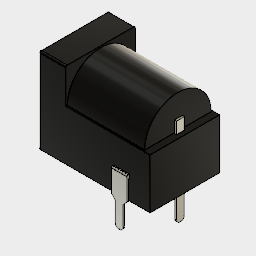
373 Breadboard Friendly 2.1 mm Barrel Jack (Autodesk Fusion 360 design; units mm, degrees)
Autodesk Fusion 360 part; units mm, degrees
sketch "Sketch1" plane through (0, 0, 0) normal (0, 0, 1) x (1, 0, 0)
  line L0 (0, 0) -> (0, 4.5)
  line L1 (0, 4.5) -> (-3.5, 4.5)
  line L2 (-3.5, 4.5) -> (-3.5, -4.5)
  line L3 (-3.5, -4.5) -> (0, -4.5)
  line L4 (0, -4.5) -> (0, 0)
  line L5 (0, 4.5) -> (10.9, 4.5)
  line L6 (10.9, 4.5) -> (10.9, -4.5)
  line L7 (10.9, -4.5) -> (0, -4.5)
  line L8 (0, -4.5) -> (0, 4.5)
  dimension "d1" = 4.5
  dimension "d2" = 3.5
  dimension "d3" = 9
  dimension "d4" = 10.9
  dimension "d5" = 9
  measures "d1" distance of L0.start L0.end
  measures "d2" distance of L0.end L1.end
  measures "d3" distance of L1.end L2.end
  measures "d4" distance of L0.end L5.end
  measures "d5" distance of L0.end L3.end
extrude "Extrude1" add sketch "Sketch1" along normal blind 6.5 contours L0 L4 L5 L6 L7 L8 makes body 1
extrude "Extrude2" add sketch "Sketch1" along normal blind 11 contours L0 L1 L2 L3 L4 L8 bodies 1
sketch "Sketch2" plane through (-3.5, 0, 0) normal (-1, 0, 0) x (0, -1, 0)
  line L0 (-4.5, 0) -> (4.5, 0)
  line L1 (4.5, 0) -> (4.5, 11)
  line L2 (4.5, 11) -> (-4.5, 11)
  line L3 (-4.5, 11) -> (-4.5, 0)
  line L4 (0, 11) -> (0, 0) construction
  line L5 (-4.5, 6.5) -> (4.5, 6.5) construction
  circle A0 centre (0, 6.5) radius 4.3
  circle A1 centre (0, 6.5) radius 3.25
  circle A2 centre (0, 6.472) radius 1
  dimension "d10" = 8.6
  dimension "d11" = 6.5
  dimension "d14" = 2
  measures "d10" diameter of A0
  measures "d11" diameter of A1
  measures "d14" diameter of A2
extrude "Extrude3" add sketch "Sketch2" against normal blind 13.5 contours A0 | A1 | A2 bodies 1
extrude "Extrude4" cut sketch "Sketch2" against normal blind 5 contours A1 bodies 1
sketch "Sketch3" plane through (0, 0, 0) normal (0, 0, 1) x (1, 0, 0)
  line L0 (4.325, -0.5) -> (4.075, -0.5)
  line L1 (4.075, -0.5) -> (4.075, 0.5)
  line L2 (4.075, 0.5) -> (4.325, 0.5)
  line L3 (4.325, 0.5) -> (4.325, -0.5)
  line L4 (4.325, -0.5) -> (4.075, 0.5) construction
  line L5 (4.075, -0.5) -> (4.325, 0.5) construction
  line L6 (3.325, 0.5) -> (3.325, -0.5)
  line L7 (-3.5, 4.5) -> (-3.5, -4.5)
  line L8 (10.325, -0.5) -> (10.075, -0.5)
  line L9 (10.075, -0.5) -> (10.075, 0.5)
  line L10 (10.075, 0.5) -> (10.325, 0.5)
  line L11 (10.325, 0.5) -> (10.325, -0.5)
  line L12 (10.325, -0.5) -> (10.075, 0.5) construction
  line L13 (10.075, -0.5) -> (10.325, 0.5) construction
  point P0 (4.2, 0)
  point P1 (10.2, 0)
  dimension "d17" = 0.25
  dimension "d18" = 1
  dimension "d19" = 1
  dimension "d20" = 7.7
  dimension "d21" = 1
  dimension "d22" = 0.25
  dimension "d23" = 6
  measures "d17" distance of L1.end L2.end
  measures "d18" distance of L0.end L1.end
  measures "d19" distance of L3
  measures "d20" distance of P0 L7
  measures "d21" distance of L8.end L9.end
  measures "d22" distance of L9.end L10.end
  measures "d23" distance of P0 P1
extrude "Extrude11" cut sketch "Sketch3" along normal blind 10 contours L8 L9 L10 L11 bodies 1
extrude "Extrude5" add sketch "Sketch3" along normal blind 8 and the other way blind 3.5 separate body makes body 2 at (4.325, -0.1667, 4.1667) makes body 3 at (10.325, -0.1667, 4.1667)
sketch "Sketch4" plane through (0, -4.5, 0) normal (0, -1, 0) x (1, 0, 0)
  line L0 (-3.5, 0) -> (10.9, 0)
  line L1 (10.9, 0) -> (10.9, 6.5)
  line L2 (10.9, 6.5) -> (0, 6.5)
  line L3 (0, 6.5) -> (0, 11)
  line L4 (0, 11) -> (-3.5, 11)
  line L5 (-3.5, 11) -> (-3.5, 0)
  line L6 (8.2, 3) -> (6.2, 3)
  line L7 (6.2, 3) -> (6.2, 0)
  line L8 (6.2, 0) -> (8.2, 0)
  line L9 (8.2, 0) -> (8.2, 3)
  line L10 (8.2, 3) -> (6.2, 0) construction
  line L11 (6.2, 3) -> (8.2, 0) construction
  line L12 (-3.5, 11) -> (-3.5, 0)
  line L13 (10.9, 0) -> (0, 0)
  point P0 (7.2, 1.5)
  dimension "d26" = 2
  dimension "d27" = 3
  dimension "d28" = 10.7
  dimension "d29" = 1.5
  measures "d26" distance of L7.end L8.end
  measures "d27" distance of L6.end L7.end
  measures "d28" distance of P0 L12
  measures "d29" distance of P0 L13
extrude "Extrude6" add sketch "Sketch4" along normal blind 0.3 separate body contours L0 L6 L7 L8 L9 L13 makes body 4
sketch "Sketch5" plane through (0, 0, 0) normal (0, 0, -1) x (1, 0, 0)
  line L0 (6.2, 4.6) -> (8.2, 4.6)
  line L1 (6.2, 4.5) -> (8.2, 4.5)
  line L2 (8.2, 4.5) -> (8.2, 4.8)
  line L3 (8.2, 4.8) -> (6.2, 4.8)
  line L4 (6.2, 4.8) -> (6.2, 4.5)
extrude "Extrude10" cut sketch "Sketch5" against normal blind 2.5 contours L0 L1 L2 L4 bodies 4
extrude "Extrude8" add 1 faces at (7.5333, -4.7333, 0) along direction (0, 0, -1) blind 3.5 on bodies 4 bodies 4
sketch "Sketch6" plane through (0, -4.8, 0) normal (0, -1, 0) x (1, 0, 0)
  line L0 (8.2, -3.5) -> (8.2, 3)
  line L1 (8.2, 3) -> (6.2, 3)
  line L2 (6.2, 3) -> (6.2, -3.5)
  line L3 (6.2, -3.5) -> (8.2, -3.5)
  line L4 (7.7, 0) -> (6.7, 0)
  line L5 (6.7, 0) -> (6.7, -3.5)
  line L6 (6.7, -3.5) -> (7.7, -3.5)
  line L7 (7.7, -3.5) -> (7.7, 0)
  line L8 (7.7, 0) -> (6.7, -3.5) construction
  line L9 (6.7, 0) -> (7.7, -3.5) construction
  line L10 (6.2, 0) -> (6.7126, -0.5126)
  line L11 (8.2, -0.0002) -> (7.6389, -0.5613)
  line L12 (8.2, -0.0002) -> (8.9935, -0.0002) construction
  point P0 (7.2, -1.75)
  dimension "d36" = 1
  dimension "d37" = 3.5
  dimension "d38" = 1.75
  dimension "d39" = 1
  dimension "d41" = 135
  measures "d36" distance of L5.end L6.end
  measures "d37" distance of L4.end L5.end
  measures "d38" distance of L3 P0
  measures "d39" distance of L0 P0
  measures "d41" angle of L11 L12
extrude "Extrude9" cut sketch "Sketch6" against normal up to surface (0.2 mm away) contours L0 L3 L7 L11 | L2 L3 L5 L10 bodies 4
fillet "Fillet1" radius 0.4 6 edges at (4.2, -0.5, -3.5) (4.2, 0.5, -3.5) (10.2, -0.5, -3.5) (10.2, 0.5, -3.5) (7.7, -4.7, -3.5) (6.7, -4.7, -3.5) on bodies 2 3 4
fillet "Fillet2" radius 1 1 edges at (-3.5, 0.9323, 6.1104) on bodies 1
fillet "Fillet3" radius 0.2 6 edges at (-3.5, 0, 11) (-3.5, -4.5, 5.5) (-3.5, 4.5, 5.5) (-3.5, 0, 0) (-1.75, 4.5, 11) (-1.75, -4.5, 11) on bodies 1
fillet "Fillet4" radius 0.15 1 edges at (7.2, -4.8, 3) on bodies 4
equation "d4 = 14.4 mm - 3.5 mm"
equation "d20 = 10.7 mm - 3 mm"
equation "d38 = ( 3.5 / 2 ) * 1 mm"
